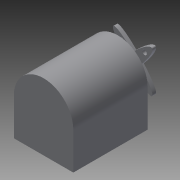
# Autodesk Inventor part: servo
Saved by Autodesk Inventor 2014 (Build 180170000, 170)
## iProperties
Created: 2014-11-30
Part Number: servo
Material: Aluminum 6061, Welded
Document SubType Name: Modeling
Designer: ph1140784
Density: 2.71 g/cm^3
Appearance: Weld - Aluminum
Mass: 224.292 g
Surface Area: 121.925 cm^2
Volume: 82.7644 cm^3
Author: ph1140784
Autodesk Inventor part; units mm, degrees
ref_plane "YZ Plane" through (0, 0, 0) normal (1, 0, 0) x (0, 1, 0)
ref_plane "XZ Plane" through (0, 0, 0) normal (0, 1, 0) x (-1, 0, 0)
ref_plane "XY Plane" through (0, 0, 0) normal (0, 0, 1) x (1, 0, 0)
sketch "Sketch1" plane through (0, 0, 0) normal (0, 1, 0) x (-1, 0, 0)
  arc A0 (20, 9.3923) -> (-20, 9.3923) centre (0, 9.3923) ccw
  line L0 (-20, -15.6077) -> (20, -15.6077)
  line L1 (20, -15.6077) -> (20, 9.3923)
  line L2 (-20, 9.3923) -> (-20, -15.6077)
  point P0 (0, 0)
  dimension "d0" = 40
  constraints: 6 end point, 2 point on circle, 2 tangent, 1 centre point
  measures "d0" diameter of A0
extrude "Extrusion1" add sketch "Sketch1" along normal blind 50
sketch "Sketch2" plane through (0, 50, 0) normal (0, 1, 0) x (1, 0, 0)
  arc A0 (-20, -9.3923) -> (20, -9.3923) centre (0, -9.3923) ccw projected
  circle A1 centre (0, -9.3923) radius 3.75
  point P0 (0, 0)
  dimension "d4" = 7.5
  constraints: 1 centre point, 1 coincident
  measures "d4" diameter of A1
extrude "Extrusion2" add sketch "Sketch2" along normal blind 10
sketch "Sketch3" plane through (0, 60, 9.3923) normal (0, 1, 0) x (1, 0, 0)
  circle A0 centre (0, 0) radius 3.75 projected
  ellipse E0 centre (0, 0) end of major axis (-13, -14) minor radius 3.6924 (-2.25, 3) -> (-3.1582, 2.0219) ccw
  ellipse E1 centre (0, 0) end of major axis (13, -14) minor radius 3.7302 (-3, -2.25) -> (-2.4658, -2.8253) ccw
  ellipse E2 centre (0, 0) end of major axis (-13, -14) minor radius 3.6924 (-4.9841, -0.0284) -> (-0.0262, -5.3386) ccw
  ellipse E3 centre (0, 0) end of major axis (-13, -14) minor radius 3.6924 (2.25, -3) -> (3.1582, -2.0219) ccw
  ellipse E4 centre (0, 0) end of major axis (-13, -14) minor radius 3.6924 (4.9841, 0.0284) -> (0.0262, 5.3386) ccw
  ellipse E5 centre (0, 0) end of major axis (13, -14) minor radius 3.7302 (-0.0262, -5.3386) -> (4.9841, 0.0284) ccw
  ellipse E6 centre (0, 0) end of major axis (13, -14) minor radius 3.7302 (3, 2.25) -> (2.4658, 2.8253) ccw
  ellipse E7 centre (0, 0) end of major axis (13, -14) minor radius 3.7302 (0.0262, 5.3386) -> (-4.9841, -0.0284) ccw
  line L0 (8, 9) -> (-8, -9) construction
  line L1 (-8, 9) -> (8, -9) construction
  circle A1 centre (-8, 9) radius 1.5
  circle A2 centre (8, 9) radius 1.5
  circle A3 centre (8, -9) radius 1.5
  circle A4 centre (-8, -9) radius 1.5
  point P0 (0, 9.3923)
  dimension "d7" = 3
  dimension "d8" = 3
  dimension "d9" = 3
  dimension "d10" = 3
  constraints: 6 coincident, 4 centre point, 4 end point, 2 midpoint, 41 other
  measures "d7" diameter of A1
  measures "d8" diameter of A2
  measures "d9" diameter of A3
  measures "d10" diameter of A4
extrude "Extrusion3" add sketch "Sketch3" along normal blind 2.5
sketch "Sketch4" plane through (0, 60, 9.3923) normal (0, 1, 0) x (1, 0, 0)
  circle A0 centre (0, 0) radius 3.75 projected
  point P0 (0, 9.3923)
extrude "Extrusion4" add sketch "Sketch4" along normal blind 2.5
body "Solid1"
